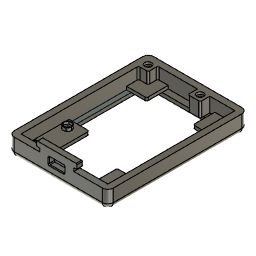
shell v1 (Autodesk Fusion 360 design; units mm, degrees)
Autodesk Fusion 360 part; units mm, degrees
note: some values were not read from the file. Set by a fixed rule: which face or edge a step refers to.
sketch "草图1" plane through (0, 0, 0) normal (0, 0, 1) x (1, 0, 0)
  line L0 (-4, -4) -> (60, -4)
  line L1 (60, -4) -> (60, 86)
  line L2 (60, 86) -> (-4, 86)
  line L3 (-4, 86) -> (-4, -4)
  dimension "d1" = 64
  dimension "d2" = 90
  constraint horizontal L0
  constraint vertical L1
  constraint horizontal L2
  constraint vertical L3
  measures "d1" distance of L0.start L0.end
  measures "d2" distance of L0.start L2.end
extrude "拉伸1" add sketch "草图1" along normal blind 11.65
sketch "草图2" plane through (0, 0, 11.65) normal (0, 0, 1) x (-1, 0, 0)
  line L0 (4, -86) -> (4, 4)
  line L1 (4, 4) -> (-60, 4)
  line L2 (-60, 4) -> (-60, -86)
  line L3 (-60, -86) -> (4, -86)
shell "抽壳1" thickness 4 removed faces 1 at (17.3333, 56, 11.65)
move_face "偏移面1" offset -1.7 1 faces at (18.6667, 27.3333, 4)
sketch "草图3" plane through (0, 0, 0) normal (0, 0, 1) x (1, 0, 0)
  line L0 (3, 8.8) -> (53, 8.8)
  line L1 (53, 8.8) -> (53, 78)
  line L2 (53, 78) -> (3, 78)
  line L3 (3, 78) -> (3, 8.8)
  dimension "d7" = 50
  dimension "d8" = 69.2
  constraint horizontal L0
  constraint vertical L1
  constraint horizontal L2
  constraint vertical L3
  measures "d7" distance of L0.start L0.end
  measures "d8" distance of L0.start L2.end
extrude "拉伸2" cut sketch "草图3" along normal blind 16
sketch "草图4" plane through (0, 0, 11.65) normal (0, 0, 1) x (-1, 0, 0)
sketch "草图5" plane through (0, 0, 11.65) normal (0, 0, 1) x (1, 0, 0)
sketch "草图6" plane through (0, 0, 2.3) normal (0, 0, 1) x (-1, 0, 0)
  line L0 (-3, -78) -> (-53, -78)
  line L1 (-53, -78) -> (-53, -8.8)
  line L2 (-53, -8.8) -> (-3, -8.8)
  line L3 (-3, -8.8) -> (-3, -78)
  line L4 (0, -82) -> (0, 0)
  line L5 (0, 0) -> (-56, 0)
  line L6 (-56, 0) -> (-56, -82)
  line L7 (-56, -82) -> (0, -82)
  line L8 (-56, 0) -> (-43, 0)
  line L9 (-43, 0) -> (-43, -19)
  line L10 (-43, -19) -> (-56, -19)
  line L11 (-56, -19) -> (-56, 0)
  line L12 (0, 0) -> (-13, 0)
  line L13 (-13, 0) -> (-13, -31)
  line L14 (-13, -31) -> (0, -31)
  line L15 (0, -31) -> (0, 0)
  line L16 (0, -82) -> (-13, -82)
  line L17 (-13, -82) -> (-13, -68)
  line L18 (-13, -68) -> (0, -68)
  line L19 (0, -68) -> (0, -82)
  line L20 (-56, -82) -> (-43, -82)
  line L21 (-43, -82) -> (-43, -68)
  line L22 (-43, -68) -> (-56, -68)
  line L23 (-56, -68) -> (-56, -82)
  constraint horizontal L8
  constraint vertical L9
  constraint horizontal L10
  constraint vertical L11
  constraint coincident L5.end L6.start
  constraint horizontal L12
  constraint vertical L13
  constraint horizontal L14
  constraint vertical L15
  constraint coincident L4.end L5.start
  constraint horizontal L16
  constraint vertical L17
  constraint horizontal L18
  constraint vertical L19
  constraint coincident L4.start L7.end
  constraint horizontal L20
  constraint vertical L21
  constraint horizontal L22
  constraint vertical L23
  constraint coincident L6.end L7.start
extrude "拉伸3" add sketch "草图6" along normal blind 2 contours L0 L3 L4 L7 L16 L17 L18 L19 | L0 L3 L17 L18 | L0 L1 L6 L7 L20 L21 L22 L23 | L0 L1 L21 L22 | L2 L3 L13 L14 | L2 L3 L4 L5 L12 L13 L14 L15 | L1 L2 L5 L6 L8 L9 L10 L11 | L1 L2 L9 L10
sketch "草图7" plane through (0, 0, 2.3) normal (0, 0, 1) x (-1, 0, 0)
  line L0 (-43, 0) -> (-43, -8.8)
  line L1 (-43, -8.8) -> (-13, -8.8)
  line L2 (-13, -8.8) -> (-13, 0)
  line L3 (-13, 0) -> (-43, 0)
sketch "草图8" plane through (0, 0, 4.3) normal (0, 0, 1) x (-1, 0, 0)
  line L0 (0, -31) -> (0, 0)
  line L1 (0, 0) -> (-13, 0)
  line L2 (-13, 0) -> (-13, -31)
  line L3 (-13, -31) -> (0, -31)
  circle A0 centre (-4.32, -4.3) radius 2.75
  dimension "d15" = 5.5
  measures "d15" diameter of A0
sketch "草图9" plane through (0, 0, 2.3) normal (0, 0, 1) x (-1, 0, 0)
  line L0 (-3, -68) -> (0, -68)
  line L1 (0, -68) -> (0, -31)
  line L2 (0, -31) -> (-3, -31)
  line L3 (-3, -31) -> (-3, -68)
sketch "草图10" plane through (0, 0, 4.3) normal (0, 0, 1) x (-1, 0, 0)
  line L0 (0, 0) -> (-4.32, 0)
  line L1 (-4.32, 0) -> (-4.32, -25.6)
  line L2 (-4.32, -25.6) -> (0, -25.6)
  line L3 (0, -25.6) -> (0, 0)
  circle A0 centre (-4.32, -25.6) radius 2
  circle A1 through (-50.85, -35.7, -2) (-54.975, -33.3184, -2) (-54.975, -38.0816, -2)
  line L4 (-56, -82, -2) -> (-53.66, -82, -2)
  line L5 (-53.66, -82, -2) -> (-53.66, -51.09, -2)
  line L6 (-53.66, -51.09, -2) -> (-56, -51.09, -2)
  line L7 (-56, -51.09, -2) -> (-56, -82, -2)
  circle A2 through (-50.91, -51.09, -2) (-55.035, -48.7084, -2) (-55.035, -53.4716, -2)
  line L8 (0, -82) -> (-2.2, -82)
  line L9 (-2.2, -82) -> (-2.2, -79.8)
  line L10 (-2.2, -79.8) -> (0, -79.8)
  line L11 (0, -79.8) -> (0, -82)
  line L12 (-56, -82, -2) -> (-35.8, -82, -2)
  line L13 (-35.8, -82, -2) -> (-35.8, -79.8, -2)
  line L14 (-35.8, -79.8, -2) -> (-56, -79.8, -2)
  line L15 (-56, -79.8, -2) -> (-56, -82, -2)
  dimension "d18" = 4.32
  dimension "d19" = 25.6
  dimension "d20" = 4
  dimension "d23" = 5.5
  dimension "d24" = 2.34
  dimension "d25" = 30.91
  dimension "d26" = 5.5
  dimension "d27" = 2.2
  dimension "d28" = 2.2
  dimension "d29" = 20.2
  dimension "d30" = 2.2
  constraint horizontal L0
  constraint vertical L1
  constraint horizontal L2
  constraint vertical L3
  constraint coincident L0.start L3.end
  constraint coincident L1.end L2.start
  constraint horizontal L8
  constraint vertical L9
  constraint horizontal L10
  constraint vertical L11
  measures "d18" distance of L0.start L0.end
  measures "d19" distance of L0.start L2.end
  measures "d20" diameter of A0
  measures "d27" distance of L8.start L8.end
  measures "d28" distance of L8.start L10.end
sketch "草图11" plane through (0, 0, 2.3) normal (0, 0, 1) x (-1, 0, 0)
  line L0 (-13, -82) -> (-13, -78)
  line L1 (-13, -78) -> (-43, -78)
  line L2 (-43, -78) -> (-43, -82)
  line L3 (-43, -82) -> (-13, -82)
  line L4 (-31.8, -82) -> (-39.8, -82)
  line L5 (-39.8, -82) -> (-39.8, -75.8)
  line L6 (-39.8, -75.8) -> (-31.8, -75.8)
  line L7 (-31.8, -75.8) -> (-31.8, -82)
  line L8 (-56, -51.09) -> (-56, -82)
  dimension "d31" = 8
  dimension "d32" = 6.2
  dimension "d34" = 16.2
  dimension "d35" = 6.2
  constraint horizontal L4
  constraint vertical L5
  constraint horizontal L6
  constraint vertical L7
  measures "d31" distance of L4.start L4.end
  measures "d32" distance of L4.start L6.end
  measures "d34" distance of L5 L8
  measures "d35" distance of L3 L6
sketch "草图12" plane through (0, 0, 4.3) normal (0, 0, 1) x (-1, 0, 0)
  line L0 (0, -68) -> (-13, -68)
  line L1 (-13, -68) -> (-13, -82)
  line L2 (-13, -82) -> (0, -82)
  line L3 (0, -82) -> (0, -68)
  line L4 (0, -82) -> (-6.2, -82)
  line L5 (-6.2, -82) -> (-6.2, -75.8)
  line L6 (-6.2, -75.8) -> (0, -75.8)
  line L7 (0, -75.8) -> (0, -82)
  dimension "d36" = 6.2
  dimension "d37" = 6.2
  constraint horizontal L4
  constraint vertical L5
  constraint horizontal L6
  constraint vertical L7
  constraint coincident L2.end L3.start
  measures "d36" distance of L2.end L4.end
  measures "d37" distance of L2.end L6.end
extrude "拉伸4" add sketch "草图11" along normal blind 9.35 contours L1 L3 L4 L5 L7 | L1 L5 L6 L7
extrude "拉伸5" add sketch "草图12" along normal blind 7.35 contours L2 L3 L4 L5 L6 L7
extrude "拉伸6" add sketch "草图10" along normal blind 4 contours A1 | L5 L6 L7 A2 | L5 L6 L7 A2 in plane through (0, 0, 2.3) normal (0, 0, 1)
extrude "拉伸7" add sketch "草图8" along normal blind 2 contours A0
sketch "草图13" plane through (0, 0, 4.3) normal (0, 0, 1) x (-1, 0, 0)
  circle A0 centre (-4.32, -4.3) radius 2.75
  line L0 (0, -31) -> (0, 0)
  line L1 (0, 0) -> (-13, 0)
  line L2 (-13, 0) -> (-13, -31)
  line L3 (-13, -31) -> (0, -31)
  line L4 (0, 0) -> (-4.32, 0)
  line L5 (-4.32, 0) -> (-4.32, -25.6)
  line L6 (-4.32, -25.6) -> (0, -25.6)
  line L7 (0, -25.6) -> (0, 0)
  circle A1 centre (-4.32, -25.6) radius 2.75
  dimension "d46" = 4.32
  dimension "d47" = 25.6
  dimension "d48" = 5.5
  constraint horizontal L4
  constraint vertical L5
  constraint horizontal L6
  constraint vertical L7
  constraint coincident L0.end L1.start
  constraint coincident L5.end L6.start
  measures "d46" distance of L0.end L4.end
  measures "d47" distance of L0.end L6.end
  measures "d48" diameter of A1
extrude "拉伸8" add sketch "草图13" along normal blind 2 contours L5 L6 A1 | L5 L6 A1
sketch "草图14" plane through (0, 0, 11.65) normal (0, 0, 1) x (-1, 0, 0)
  line L0 (-6.2, -82) -> (-31.8, -82)
  line L1 (-31.8, -82) -> (-31.8, -75.8)
  line L2 (-31.8, -75.8) -> (-39.8, -75.8)
  line L3 (-39.8, -75.8) -> (-39.8, -82)
  line L4 (-39.8, -82) -> (-56, -82)
  line L5 (-56, -82) -> (-56, 0)
  line L6 (-56, 0) -> (0, 0)
  line L7 (0, 0) -> (0, -75.8)
  line L8 (0, -75.8) -> (-6.2, -75.8)
  line L9 (-6.2, -75.8) -> (-6.2, -82)
  line L10 (4, -86) -> (4, 4)
  line L11 (4, 4) -> (-60, 4)
  line L12 (-60, 4) -> (-60, -86)
  line L13 (-60, -86) -> (4, -86)
  line L14 (0, -82) -> (-2.2, -82)
  line L15 (-2.2, -82) -> (-2.2, -79.8)
  line L16 (-2.2, -79.8) -> (0, -79.8)
  line L17 (0, -79.8) -> (0, -82)
  dimension "d51" = 2.2
  dimension "d52" = 2.2
  constraint horizontal L14
  constraint vertical L15
  constraint horizontal L16
  constraint vertical L17
  measures "d51" distance of L14.start L14.end
  measures "d52" distance of L14.start L16.end
hole "孔1" at (2.2, 79.8, 11.65) direction (0, 0, -1) diameter 2 depth 7 tip angle 118 counterbore diameter 4.5 counterbore depth 1.5
sketch "草图15" plane through (0, 0, 11.65) normal (0, 0, 1) x (-1, 0, 0)
  circle A0 centre (-2.2, -79.8) radius 2.25
  line L0 (-6.2, -82) -> (-31.8, -82)
  line L1 (-31.8, -82) -> (-31.8, -75.8)
  line L2 (-31.8, -75.8) -> (-39.8, -75.8)
  line L3 (-39.8, -75.8) -> (-39.8, -82)
  line L4 (-39.8, -82) -> (-56, -82)
  line L5 (-56, -82) -> (-56, 0)
  line L6 (-56, 0) -> (0, 0)
  line L7 (0, 0) -> (0, -75.8)
  line L8 (0, -75.8) -> (-6.2, -75.8)
  line L9 (-6.2, -75.8) -> (-6.2, -82)
  line L10 (4, -86) -> (4, 4)
  line L11 (4, 4) -> (-60, 4)
  line L12 (-60, 4) -> (-60, -86)
  line L13 (-60, -86) -> (4, -86)
  line L14 (-56, -82) -> (-35.8, -82)
  line L15 (-35.8, -82) -> (-35.8, -79.8)
  line L16 (-35.8, -79.8) -> (-56, -79.8)
  line L17 (-56, -79.8) -> (-56, -82)
  dimension "d58" = 20.2
  dimension "d59" = 2.2
  constraint horizontal L14
  constraint vertical L15
  constraint horizontal L16
  constraint vertical L17
  constraint coincident L4.end L5.start
  measures "d58" distance of L4.end L14.end
  measures "d59" distance of L4.end L16.end
hole "孔2" at (35.8, 79.8, 11.65) direction (0, 0, -1) diameter 2 depth 7 tip angle 118 counterbore diameter 4.5 counterbore depth 1.5
sketch "草图16" plane through (0, 0, 6.3) normal (0, 0, 1) x (-1, 0, 0)
  line L0 (-56, -34.3574) -> (-56, -37.0426)
  arc A0 (-56, -37.0426) -> (-56, -34.3574) centre (-53.6, -35.7) ccw
  line L1 (-53.6, -38.45) -> (-53.6, -32.95)
  constraint coincident A0 L1.start
  constraint coincident A0 L1.end
  constraint vertical L1
sketch "草图17" plane through (0, 0, 6.3) normal (0, 0, 1) x (-1, 0, 0)
  line L0 (-56, -49.6454) -> (-56, -52.5346)
  arc A0 (-56, -52.5346) -> (-56, -49.6454) centre (-53.66, -51.09) ccw
  line L1 (-53.66, -48.34) -> (-53.66, -53.84)
  line L2 (-53.66, -48.4688) -> (-55.93, -49.7794)
  line L3 (-55.93, -49.7794) -> (-55.93, -52.4006)
  line L4 (-55.93, -52.4006) -> (-53.66, -53.7112)
  line L5 (-53.66, -53.7112) -> (-51.39, -52.4006)
  line L6 (-51.39, -52.4006) -> (-51.39, -49.7794)
  line L7 (-51.39, -49.7794) -> (-53.66, -48.4688)
  point P0 (-53.66, -51.09)
  dimension "d65" = 2.27
  constraint coincident A0 L1.start
  constraint coincident A0 L1.end
  constraint parallel L0 L1
  constraint coincident P0 A0.centre
  measures "d65" distance of P0 L7
sketch "草图18" plane through (0, 0, 6.3) normal (0, 0, 1) x (-1, 0, 0)
  line L0 (-53.5969, -32.9788) -> (-55.8684, -34.2867)
  line L1 (-55.8684, -34.2867) -> (-55.8716, -36.9079)
  line L2 (-55.8716, -36.9079) -> (-53.6031, -38.2212)
  line L3 (-53.6031, -38.2212) -> (-51.3316, -36.9133)
  line L4 (-51.3316, -36.9133) -> (-51.3284, -34.2921)
  line L5 (-51.3284, -34.2921) -> (-53.5969, -32.9788)
  point P0 (-53.6, -35.6)
  dimension "d66" = 2.27
  measures "d66" distance of P0 L5
sketch "草图19" plane through (0, 0, 6.3) normal (0, 0, 1) x (1, 0, 0)
sketch "草图20" plane through (0, 0, 6.3) normal (0, 0, 1) x (-1, 0, 0)
  circle A0 centre (-4.32, -25.6) radius 2.75
  line L0 (-5.6306, -23.33) -> (-6.9412, -25.6)
  line L1 (-6.9412, -25.6) -> (-5.6306, -27.87)
  line L2 (-5.6306, -27.87) -> (-3.0094, -27.87)
  line L3 (-3.0094, -27.87) -> (-1.6988, -25.6)
  line L4 (-1.6988, -25.6) -> (-3.0094, -23.33)
  line L5 (-3.0094, -23.33) -> (-5.6306, -23.33)
  line L6 (-5.6106, -2.03) -> (-6.9212, -4.3)
  line L7 (-6.9212, -4.3) -> (-5.6106, -6.57)
  line L8 (-5.6106, -6.57) -> (-2.9894, -6.57)
  line L9 (-2.9894, -6.57) -> (-1.6788, -4.3)
  line L10 (-1.6788, -4.3) -> (-2.9894, -2.03)
  line L11 (-2.9894, -2.03) -> (-5.6106, -2.03)
  point P0 (-4.32, -25.6)
  point P1 (-4.3, -4.3)
  dimension "d67" = 2.27
  dimension "d68" = 2.27
  constraint coincident P0 A0.centre
  measures "d67" distance of P0 L5
  measures "d68" distance of P1 L11
extrude "拉伸9" cut sketch "草图18" sketch "草图17" sketch "草图20" against normal blind 1.5 of sketch 2 contours L1 L5 L6 L7 | L1 L2 L3 L4 of sketch 3 contours L0 L1 L2 L3 L4 L5 | L6 L7 L8 L9 L10 L11
hole "孔3" at (4.32, 25.6, 4.8) direction (0, 0, -1) diameter 2 depth 7 tip angle 118
hole "孔4" at (4.3, 4.3, 4.8) direction (0, 0, -1) diameter 2 depth 4 tip angle 180
hole "孔5" at (53.6, 35.7, 6.3) direction (0, 0, -1) diameter 2 depth 4 tip angle 180
hole "孔6" at (53.66, 51.09, 4.8) direction (0, 0, -1) diameter 2 depth 2.5 tip angle 180
sketch "草图21" plane through (0, 0, 2.3) normal (0, 0, 1) x (-1, 0, 0)
  arc A0 (-56, -37.0426) -> (-53, -38.3837) centre (-53.6, -35.7) ccw
  line L0 (-56, -37.0426) -> (-56, -49.6454)
  arc A1 (-53, -48.4204) -> (-56, -49.6454) centre (-53.66, -51.09) ccw
  line L1 (-53, -48.4204) -> (-53, -38.3837)
  line L2 (-56, -49.6454) -> (-52, -49.6454)
  line L3 (-52, -49.6454) -> (-52, -37)
  line L4 (-52, -37) -> (-56, -37)
  line L5 (-56, -37) -> (-56, -49.6454)
  constraint horizontal L2
  constraint vertical L3
  constraint horizontal L4
  constraint vertical L5
  constraint coincident L0.end A1.end
extrude "拉伸10" add sketch "草图21" along normal blind 2 contours A0 L0 A1 L1 L5
sketch "草图22" plane through (0, -4, 0) normal (0, -1, 0) x (1, 0, 0)
  line L0 (-4, 0) -> (60, 0)
  line L1 (60, 0) -> (60, 11.65)
  line L2 (60, 11.65) -> (-4, 11.65)
  line L3 (-4, 11.65) -> (-4, 0)
  line L4 (21.84, 11.785) -> (31.84, 11.785)
  line L5 (31.84, 11.785) -> (31.84, 7.385)
  line L6 (31.84, 7.385) -> (21.84, 7.385)
  line L7 (21.84, 7.385) -> (21.84, 11.785)
  line L8 (14.5107, 16.95) -> (39.5107, 16.95)
  line L9 (40.0107, 16.45) -> (40.0107, 13.95)
  line L10 (40.0107, 13.95) -> (14.0107, 13.95)
  line L11 (14.0107, 13.95) -> (14.0107, 16.45)
  line L12 (38.0107, 13.95) -> (16.0107, 13.95)
  line L13 (16.0107, 13.95) -> (16.0107, 13.65)
  line L14 (16.0107, 13.65) -> (38.0107, 13.65)
  line L15 (38.0107, 13.65) -> (38.0107, 13.95)
  line L16 (16.0107, 13.65) -> (38.0107, 13.65)
  line L17 (38.0107, 13.65) -> (38.0107, 11.65)
  line L18 (38.0107, 11.65) -> (16.0107, 11.65)
  line L19 (16.0107, 11.65) -> (16.0107, 13.65)
  line L20 (14.0107, 13.95) -> (16.0107, 13.65)
  line L21 (40.0107, 13.95) -> (38.0107, 13.65)
  arc A0 (14.5107, 16.95) -> (14.0107, 16.45) centre (14.5107, 16.45) ccw
  line L22 (88, 25) -> (88, 22)
  line L23 (88, 22) -> (86, 21.7)
  line L24 (88, 22) -> (62, 22)
  line L25 (86, 22) -> (64, 22)
  line L26 (62.5, 25) -> (88, 25)
  line L27 (62, 22) -> (64, 21.7)
  line L28 (86, 19.7) -> (64, 19.7)
  line L29 (64, 21.7) -> (86, 21.7)
  line L30 (62, 22) -> (62, 24.5)
  line L31 (64, 21.7) -> (86, 21.7)
  line L32 (86, 21.7) -> (86, 22)
  line L33 (64, 22) -> (64, 21.7)
  line L34 (64, 19.7) -> (64, 21.7)
  arc A1 (62.5, 25) -> (62, 24.5) centre (62.5, 24.5) ccw
  line L35 (86, 21.7) -> (86, 19.7)
  arc A2 (40.0107, 16.45) -> (39.5107, 16.95) centre (39.5107, 16.45) ccw
  point P0 (14.0107, 16.95)
  point P1 (40.0107, 16.95)
  point P2 (62, 25)
  dimension "d85" = 10
  dimension "d86" = 4.4
  dimension "d87" = 7.385
  dimension "d88" = 25.84
  dimension "d89" = 26
  dimension "d90" = 3
  dimension "d91" = 22
  dimension "d92" = 0.3
  dimension "d93" = 0.3
  dimension "d94" = 22
  dimension "d95" = 2
  dimension "d96" = 0.5
  dimension "d97" = 26
  dimension "d98" = 3
  dimension "d99" = 22
  dimension "d100" = 0.3
  dimension "d101" = 0.3
  dimension "d102" = 22
  dimension "d103" = 2
  dimension "d104" = 0.5
  dimension "d105" = 0.5
  constraint horizontal L4
  constraint vertical L5
  constraint horizontal L6
  constraint vertical L7
  constraint horizontal L8
  constraint vertical L9
  constraint horizontal L10
  constraint vertical L11
  constraint horizontal L12
  constraint vertical L13
  constraint horizontal L14
  constraint vertical L15
  constraint horizontal L16
  constraint vertical L17
  constraint horizontal L18
  constraint vertical L19
  constraint coincident P0 L8
  constraint coincident P0 L11
  constraint tangent L8 A0
  constraint tangent L11 A0
  constraint horizontal L26
  constraint vertical L22
  constraint horizontal L24
  constraint vertical L30
  constraint horizontal L25
  constraint vertical L33
  constraint horizontal L31
  constraint vertical L32
  constraint horizontal L29
  constraint vertical L35
  constraint horizontal L28
  constraint vertical L34
  constraint coincident P2 L26
  constraint coincident P2 L30
  constraint tangent L26 A1
  constraint tangent L30 A1
  constraint coincident P1 L8
  constraint coincident P1 L9
  constraint tangent L8 A2
  constraint tangent L9 A2
  constraint coincident L2 L17.end
  measures "d85" distance of L4.start L4.end
  measures "d86" distance of L4.start L6.end
  measures "d87" distance of L0 L6
  measures "d88" distance of L3 L7
  measures "d89" distance of P0 P1
  measures "d90" distance of P0 L10.end
  measures "d91" distance of L12.start L12.end
  measures "d92" distance of L12.start L14.end
  measures "d93" distance of L10 L14
  measures "d94" distance of L13.end L14.end
  measures "d95" distance of L13.end L18.end
  measures "d96" radius of A0
  measures "d97" distance of L22.start P2
  measures "d98" distance of P2 L24.end
  measures "d99" distance of L25.end L25.start
  measures "d100" distance of L23.end L25.start
  measures "d101" distance of L24 L31
  measures "d102" distance of L27.end L23.end
  measures "d103" distance of L27.end L28.end
  measures "d104" radius of A1
  measures "d105" radius of A2
extrude "拉伸11" add sketch "草图22" against normal blind 4 contours L2 L4 L5 L7 L14 L16 L17 L18 L19 | L10 L13 L20 | L10 L12 L13 L14 L15 L16 | L10 L15 L21 | L8 L9 L10 L11 L12 A0 A2
extrude "拉伸12" cut 1 faces at (28.5067, -1.3333, 11.65) along direction (0, 0, -1) blind 4.265
fillet "圆角1" radius 3.5 1 edges at (-4, -4, 5.825)
fillet "圆角2" radius 3.5 1 edges at (60, -4, 5.825)
fillet "圆角3" radius 3.5 8 edges at (60, 86, 5.825) (-4, 86, 5.825) (28, 86, 0) (-4, 42.75, 0) (-2.9749, -2.9749, 0) (28, -4, 0) (58.9749, -2.9749, 0) (60, 42.75, 0)
fillet "圆角4" radius 0.5 4 faces at (25.1733, -2.6667, 11.785) (21.84, -2.6667, 10.3183) (28.5067, -1.3333, 7.385) (31.84, -1.3333, 8.8517)
fillet "圆角5" radius 1 9 edges at (13, 68, 3.3) (43, 68, 3.3) (13, 31, 3.3) (43, 19, 3.3) (31.8, 75.8, 6.975) (6.2, 75.8, 7.975) (39.8, 75.8, 6.975) (6.2, 82, 7.975) (0, 75.8, 7.975)
fillet "圆角6" radius 0.5 9 edges at (38.0107, 0, 12.65) (39.0107, 0, 13.8) (14.0107, 0, 15.2) (14.1572, 0, 16.8036) (27.0107, 0, 16.95) (39.8643, 0, 16.8036) (40.0107, 0, 15.2) (15.0107, 0, 13.8) (16.0107, 0, 12.65)
